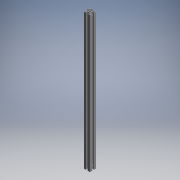
# Autodesk Inventor part: NFS5-2020-437-Z6-XA10-XB427
Saved by Autodesk Inventor 2017.3 (Build 213256000, 256)
## iProperties
Part Number: NFS5-2020-437-Z6-XA10-XB427
Material: Generic
Catalog Web Link: www.cadenas.de
Description: NFS5-2020, NFSB5-2020, HFS5-2020, HFSB5-2020, CAF5-2020, HFSY5-2020, NFSF5-2020, HFSF5-2020, HFSFB5-2020, NFST5-2020, HFST5-2020, HFSTB5-2020, HFSH5-2020, HFSC5-2020-HFS5 Series Aluminum Extrusions 20 Square -1 Slot-
Vendor: MISUMI
Document SubType Name: Modeling
Designer: partserver
Manufacturer: MISUMI
Mass: 78.6573 g
Surface Area: 763.15 cm^2
Volume: 78.6573 cm^3
Density: 1 g/cm^3
Appearance: PSOLRGB-175-175-175
Category: PARTsolutions
Company: MISUMI
Title: NFS5-2020-437-Z6-XA10-XB427
Author: Cadenas PARTsolutions
Comments: HFS5 Series Aluminum Extrusions 20 Square -1 Slot-
PSOL_IDENT_0: {$CADENAS_DATA\23d-libs\misumi\metric\38_al_extrusions_blackets\5\hfs5_2020.prj},704 {VTYP=3D},{NB=N
PSOL_IDENT_1: FS5-2020-437-Z6-XA10-XB427},{LINA=NFS5-2020-437-Z6-XA10-XB427},{NN=NFS5-2020, NFSB5-2020, HFS5-2020,
PSOL_IDENT_2: HFSB5-2020, CAF5-2020, HFSY5-2020, NFSF5-2020, HFSF5-2020, HFSFB5-2020, NFST5-2020, HFST5-2020, HFS
PSOL_IDENT_3: TB5-2020, HFSH5-2020, HFSC5-2020},{DATE=09.09.2019 15:28:27},{GEOMDATE=18.06.2019 07:59:14},{VERSION=
PSOL_IDENT_4: },{LINEID=10},{WBVAR=L,ALT1,ALT2,ALT4,ALT5,CP5,DL5,DR5,ALT6,ALT9,ALT10,ALT11,HP6,NHL6,DL6,NHR6,DR6,A
PSOL_IDENT_5: LT7,ALT8,NH9,AH,BH,CH,DH,EH,NH10,AV,BV,CV,DV,EV,NH11,AP,BP,CP,DP,EP,ALT12,ALT13,Z,NH12,XA,XB,XC,XD,X
PSOL_IDENT_6: E,NH13,YA,YB,YC,YD,YE,ALT16,HP16,DL16,DR16,ALT17,HQ17,JLP,ALT20},{WBNUMERIC=L,NH9,AH,BH,CH,DH,EH,NH1
PSOL_IDENT_7: 0,AV,BV,CV,DV,EV,NH11,AP,BP,CP,DP,EP,NH12,XA,XB,XC,XD,XE,NH13,YA,YB,YC,YD,YE,HQ17,JLP}  {NB=NFS5-202
PSOL_IDENT_8: 0-437-Z6-XA10-XB427},{LINA=NFS5-2020-437-Z6-XA10-XB427},{KT=DUMMY},{PN=NFS5-2020-437-Z6-XA10-XB427},
PSOL_IDENT_9: {TPS=NFS5-2020},{MAT=6063-T5 Aluminum Alloy},{ST=Clear Anodize},{FRMW=20},{FRMH=20},{FRD=4.2},{L=437
PSOL_IDENT_10: },{MASS=0.5},{SA=183},{LX=0.742x10^4},{LY=0.742x10^4},{ALT1=},{M1=0},{DPL1=0},{DPR1=0},{ALT1PN=},{AL
PSOL_IDENT_11: T2=},{ALT2ALG= '','w/o End Tapping (Heli-Coil Insert)','LHP','with LHP (Tapping on the Left (Heli-Co
PSOL_IDENT_12: il Insert))','RHP','with RHP (Tapping on the Right (Heli-Coil Insert))','HPW','with HPW (Tapping on
PSOL_IDENT_13: Both Ends (Heli-Coil Insert))' },{M2=0},{DP2=0},{ALT2PN=},{ALT4=},{ALT4ALG= '', 'w/o SC (High Precis
PSOL_IDENT_14: ion Cut)', 'SC', 'with SC (High Precision Cut)' },{ALT4PN=},{ALT5=},{ALT5ALG= '','w/o 45 Degree Cut'
PSOL_IDENT_15: ,'1','with 45 Degree Cut' },{CP5=},{CP5ALG= '','N/A' },{DL5=},{DL5ALG= '','N/A' },{DR5=},{DR5ALG= ''
PSOL_IDENT_16: ,'N/A' },{FRMLALT5=0},{FRMRALT5=0},{ALT5PN=},{ALT6=},{ALT6ALG= '','w/o Fastening Location Wrench Acc
PSOL_IDENT_17: ess Hole Alterations','1','with Fastening Location Wrench Access Hole Alterations' },{ALT9=},{ALT9AL
PSOL_IDENT_18: G= '','w/o Location Specified Wrench Access Hole Alteratons (Horizontal)','1','with Location Specifi
PSOL_IDENT_19: ed Wrench Access Hole Alteratons (Horizontal)' },{ALT10=},{ALT10ALG= '','w/o Location Specified Wren
PSOL_IDENT_20: ch Access Hole Alteratons (Vertical)','1','with Location Specified Wrench Access Hole Alteratons (Ve
PSOL_IDENT_21: rtical)' },{ALT11=},{ALT11ALG= '','w/o Location Specified Wrench Access Hole Alteratons (Crisscross)'
PSOL_IDENT_22: ,'1','with Location Specified Wrench Access Hole Alteratons (Crisscross)' },{HP6=},{HP6ALG= '','N/A'
PSOL_IDENT_23: },{NHL6=},{NHL6ALG= '','N/A' },{DL6=},{DL6ALG= '','N/A' },{NHR6=},{NHR6ALG= '','N/A' },{DR6=},{DR6A
PSOL_IDENT_24: LG= '','N/A' },{HL6=0.000},{HL6D=0},{HR6=0.000},{HR6D=0},{J6=0},{J6D=0},{K6=0},{K6D=0},{DD6=0.00},{D
PSOL_IDENT_25: D6ALG=0},{ALT7=},{ALT7ALG= '','N/A' },{ALT8=},{ALT8ALG= '','N/A' },{ALT678PN=},{NH9=0},{NH9MAX=5},{N
PSOL_IDENT_26: H9ALG=[0]},{AH=0.0},{AHMIN=7},{AHMAX=432},{AHALG=[0]},{BH=0.0},{BHMIN=2},{BHMAX=434},{BHALG=[0]},{CH=
PSOL_IDENT_27: 0.0},{CHMIN=2},{CHMAX=436},{CHALG=[0]},{DH=0.0},{DHMIN=2},{DHMAX=438},{DHALG=[0]},{EH=0.0},{EHMIN=2}
PSOL_IDENT_28: ,{EHMAX=430},{EHALG=[0]},{NH10=0},{NH10MAX=5},{NH10ALG=[0]},{AV=0.0},{AVMIN=7},{AVMAX=432},{AVALG=[0
PSOL_IDENT_29: ]},{BV=0.0},{BVMIN=2},{BVMAX=434},{BVALG=[0]},{CV=0.0},{CVMIN=2},{CVMAX=436},{CVALG=[0]},{DV=0.0},{D
PSOL_IDENT_30: VMIN=2},{DVMAX=438},{DVALG=[0]},{EV=0.0},{EVMIN=2},{EVMAX=430},{EVALG=[0]},{NH11=0},{NH11MAX=5},{NH1
PSOL_IDENT_31: 1ALG=[0]},{AP=0.0},{APMIN=7},{APMAX=432},{APALG=[0]},{BP=0.0},{BPMIN=2},{BPMAX=434},{BPALG=[0]},{CP=
PSOL_IDENT_32: 0.0},{CPMIN=2},{CPMAX=436},{CPALG=[0]},{DP=0.0},{DPMIN=2},{DPMAX=438},{DPALG=[0]},{EP=0.0},{EPMIN=2}
PSOL_IDENT_33: ,{EPMAX=430},{EPALG=[0]},{ALT9PN=},{ALT10PN=},{ALT11PN=},{ALT91011PN=},{ALT12=1},{ALT12ALG= '','w/o
PSOL_IDENT_34: Counterbore Hole in Specified Position (Vertical)','1','with Counterbore Hole in Specified Position
PSOL_IDENT_35: (Vertical)' },{ALT13=},{ALT13ALG= '','w/o Counterbore Hole in Specified Position (Horizontal)','1','
PSOL_IDENT_36: with Counterbore Hole in Specified Position (Horizontal)' },{Z=6},{ZALG='5','5','6','6'},{DD12=6.5},
PSOL_IDENT_37: {DD112=11.0},{NH12=2},{NH12MAX=5},{NH12ALG=[1:5/1]},{XA=10.0},{XAMIN=7},{XAMAX=417},{XAALG=[7:417/0.
PSOL_IDENT_38: 5]},{XB=427.0},{XBMIN=23},{XBMAX=430},{XBALG=[23:430/0.5]},{XC=0.0},{XCMIN=440},{XCMAX=443},{XCALG=[
PSOL_IDENT_39: 0]},{XD=0.0},{XDMIN=13},{XDMAX=456},{XDALG=[0]},{XE=0.0},{XEMIN=13},{XEMAX=430},{XEALG=[0]},{NH13=0}
PSOL_IDENT_40: ,{NH13MAX=5},{NH13ALG=[0]},{YA=0.0},{YAMIN=7},{YAMAX=443},{YAALG=[0]},{YB=0.0},{YBMIN=13},{YBMAX=456
PSOL_IDENT_41: },{YBALG=[0]},{YC=0.0},{YCMIN=13},{YCMAX=469},{YCALG=[0]},{YD=0.0},{YDMIN=13},{YDMAX=482},{YDALG=[0]
PSOL_IDENT_42: },{YE=0.0},{YEMIN=13},{YEMAX=430},{YEALG=[0]},{ALT12PN=-XA10-XB427},{ALT13PN=},{ALT1213PN=-Z6-XA10-X
PSOL_IDENT_43: B427},{ALT16=},{ALT16ALG= '','w/o M Type Hole Alteration','1','with M Type Hole Alteration' },{HP16=
PSOL_IDENT_44: },{HP16ALG= '','N/A' },{DL16=},{DL16ALG= '','N/A' },{DR16=},{DR16ALG= '','N/A' },{H116=0},{D16=0.0},
PSOL_IDENT_45: {ALT16PN=},{ALT17=},{ALT17ALG= '','w/o L Type Hole Alteration (Top)','1','with L Type Hole Alteratio
PSOL_IDENT_46: n (Top)' },{HQ17=0},{HQ17ALG=0},{JLP=0},{JLPMIN=4.9},{JLPMAX=0},{JLPALG=[0]},{L17=0},{D17=0.0},{ALT1
PSOL_IDENT_47: 7PN=},{ALT20=},{ALT20PN=},{ERRORALT01=OK},{ERRORALT02=OK},{ERRORALT05=OK},{ERRORALT06091=OK},{ERRORA
PSOL_IDENT_48: LT06092=OK},{ERRORALT06093=OK},{ERRORALT06094=OK},{ERRORALT06101=OK},{ERRORALT06102=OK},{ERRORALT061
PSOL_IDENT_49: 03=OK},{ERRORALT06104=OK},{ERRORALT06111=OK},{ERRORALT06112=OK},{ERRORALT06113=OK},{ERRORALT06114=OK
PSOL_IDENT_50: },{ERRORALT06121=OK},{ERRORALT06122=OK},{ERRORALT06123=OK},{ERRORALT06124=OK},{ERRORALT06131=OK},{ER
PSOL_IDENT_51: RORALT06132=OK},{ERRORALT06133=OK},{ERRORALT06134=OK},{ERRORALT0616=OK},{ERRORALT06171=OK},{ERRORALT
PSOL_IDENT_52: 06172=OK},{ERRORALT06173=OK},{ERRORALT0911=OK},{ERRORALT0913=OK},{ERRORALT0916=OK},{ERRORALT0917=OK}
PSOL_IDENT_53: ,{ERRORALT1011=OK},{ERRORALT1012=OK},{ERRORALT1016=OK},{ERRORALT1017=OK},{ERRORALT1112=OK},{ERRORALT
PSOL_IDENT_54: 1113=OK},{ERRORALT1116=OK},{ERRORALT1117=OK},{ERRORALT1216=OK},{ERRORALT1217=OK},{ERRORALT1316=OK},{
PSOL_IDENT_55: ERRORALT1317=OK},{ERRORALT1617=OK},{ERRORPN=},{TFW=0}
NB: NFS5-2020-437-Z6-XA10-XB427
NN: NFS5-2020, NFSB5-2020, HFS5-2020, HFSB5-2020, CAF5-2020, HFSY5-2020, NFSF5-2020, HFSF5-2020, HFSFB5-2020, NFST5-2020, HFST5-2020, HFSTB5-2020, HFSH5-2020, HFSC5-2020
NT: HFS5 Series Aluminum Extrusions 20 Square -1 Slot-
NBSYN: $PN.
LINA: NFS5-2020-437-Z6-XA10-XB427
CATALOG: Misumi
PN: NFS5-2020-437-Z6-XA10-XB427
TPS: NFS5-2020
MAT: 6063-T5 Aluminum Alloy
ST: Clear Anodize
L: 437
MASS: 0.5
SA: 183
LX: 0.742x10^4
LY: 0.742x10^4
ALT1: w/o End Tapping
M1: 0
DPL1: 0
DPR1: 0
ALT2: w/o End Tapping (Heli-Coil Insert)
M2: 0
DP2: 0
ALT4: w/o SC (High Precision Cut)
ALT5: w/o 45 Degree Cut
CP5: N/A
DL5: N/A
DR5: N/A
ALT6: w/o Fastening Location Wrench Access Hole Alterations
ALT9: w/o Location Specified Wrench Access Hole Alteratons (Horizontal)
ALT10: w/o Location Specified Wrench Access Hole Alteratons (Vertical)
ALT11: w/o Location Specified Wrench Access Hole Alteratons (Crisscross)
HP6: N/A
NHL6: N/A
DL6: N/A
NHR6: N/A
DR6: N/A
HL6D: 0
HR6D: 0
J6D: 0
K6D: 0
DD6: 0
ALT7: N/A
ALT8: N/A
NH9: 0
AH: 0
BH: 0
CH: 0
DH: 0
EH: 0
NH10: 0
AV: 0
BV: 0
CV: 0
DV: 0
EV: 0
NH11: 0
AP: 0
BP: 0
CP: 0
DP: 0
EP: 0
ALT12: with Counterbore Hole in Specified Position (Vertical)
ALT13: w/o Counterbore Hole in Specified Position (Horizontal)
Z: 6
DD12: 6.5
DD112: 11
NH12: 2
XA: 10
XB: 427
XC: 0
XD: 0
XE: 0
NH13: 0
YA: 0
YB: 0
YC: 0
YD: 0
YE: 0
ALT16: w/o M Type Hole Alteration
HP16: N/A
DL16: N/A
DR16: N/A
H116: 0
D16: 0
ALT17: w/o L Type Hole Alteration (Top)
HQ17: 0
JLP: 0
D17: 0
ALT20: w/o CW (End Face C Chamfering)
SUPPLIER: MISUMI
ARTICLENO: NFS5-2020-437-Z6-XA10-XB427
BOMINFO: NFS5-2020-437-Z6-XA10-XB427
CREATOR: CADENAS GmbH
Autodesk Inventor part; units mm, degrees
sketch "Sketch_75" plane through (0, 0, 0) normal (0, 0, 1) x (1, 0, 0)
  line L0 (-10, -3) -> (-10, -9)
  arc A0 (-10, -9) -> (-9, -10) centre (-9, -9) ccw
  line L1 (-9, -10) -> (-3, -10)
  line L2 (-3, -10) -> (-3, -8)
  line L3 (-3, -8) -> (-6, -8)
  line L4 (-6, -8) -> (-6, -7.0607)
  line L5 (-6, -7.0607) -> (-2.9393, -4)
  line L6 (-2.9393, -4) -> (-0.6536, -4)
  arc A1 (-0.6536, -4) -> (-0.4036, -3.933) centre (-0.6536, -3.5) ccw
  line L7 (-0.4036, -3.933) -> (0, -3.7)
  line L8 (0, -3.7) -> (0.4036, -3.933)
  arc A2 (0.4036, -3.933) -> (0.9036, -3.933) centre (0.6536, -3.5) ccw
  line L9 (0.9036, -3.933) -> (1.2189, -3.751)
  line L10 (1.2189, -3.751) -> (2.5, -4)
  line L11 (2.5, -4) -> (2.9393, -4)
  line L12 (2.9393, -4) -> (6, -7.0607)
  line L13 (6, -7.0607) -> (6, -8)
  line L14 (6, -8) -> (3, -8)
  line L15 (3, -8) -> (3, -10)
  line L16 (3, -10) -> (9, -10)
  arc A3 (9, -10) -> (10, -9) centre (9, -9) ccw
  line L17 (10, -9) -> (10, -3)
  line L18 (10, -3) -> (8, -3)
  line L19 (8, -3) -> (8, -6)
  line L20 (8, -6) -> (7.0607, -6)
  line L21 (7.0607, -6) -> (4, -2.9393)
  line L22 (4, -2.9393) -> (4, -0.6536)
  arc A4 (4, -0.6536) -> (3.933, -0.4036) centre (3.5, -0.6536) ccw
  line L23 (3.933, -0.4036) -> (3.7, 0)
  line L24 (3.7, 0) -> (3.933, 0.4036)
  arc A5 (3.933, 0.4036) -> (3.933, 0.9036) centre (3.5, 0.6536) ccw
  line L25 (3.933, 0.9036) -> (3.751, 1.2189)
  line L26 (3.751, 1.2189) -> (4, 2.5)
  line L27 (4, 2.5) -> (4, 2.9393)
  line L28 (4, 2.9393) -> (7.0607, 6)
  line L29 (7.0607, 6) -> (8, 6)
  line L30 (8, 6) -> (8, 3)
  line L31 (8, 3) -> (10, 3)
  line L32 (10, 3) -> (10, 9)
  arc A6 (10, 9) -> (9, 10) centre (9, 9) ccw
  line L33 (9, 10) -> (3, 10)
  line L34 (3, 10) -> (3, 8)
  line L35 (3, 8) -> (6, 8)
  line L36 (6, 8) -> (6, 7.0607)
  line L37 (6, 7.0607) -> (2.9393, 4)
  line L38 (2.9393, 4) -> (0.6536, 4)
  arc A7 (0.6536, 4) -> (0.4036, 3.933) centre (0.6536, 3.5) ccw
  line L39 (0.4036, 3.933) -> (0, 3.7)
  line L40 (0, 3.7) -> (-0.4036, 3.933)
  arc A8 (-0.4036, 3.933) -> (-0.9036, 3.933) centre (-0.6536, 3.5) ccw
  line L41 (-0.9036, 3.933) -> (-1.2189, 3.751)
  line L42 (-1.2189, 3.751) -> (-2.5, 4)
  line L43 (-2.5, 4) -> (-2.9393, 4)
  line L44 (-2.9393, 4) -> (-6, 7.0607)
  line L45 (-6, 7.0607) -> (-6, 8)
  line L46 (-6, 8) -> (-3, 8)
  line L47 (-3, 8) -> (-3, 10)
  line L48 (-3, 10) -> (-9, 10)
  arc A9 (-9, 10) -> (-10, 9) centre (-9, 9) ccw
  line L49 (-10, 9) -> (-10, 3)
  line L50 (-10, 3) -> (-8, 3)
  line L51 (-8, 3) -> (-8, 6)
  line L52 (-8, 6) -> (-7.0607, 6)
  line L53 (-7.0607, 6) -> (-4, 2.9393)
  line L54 (-4, 2.9393) -> (-4, 0.6536)
  arc A10 (-4, 0.6536) -> (-3.933, 0.4036) centre (-3.5, 0.6536) ccw
  line L55 (-3.933, 0.4036) -> (-3.7, 0)
  line L56 (-3.7, 0) -> (-3.933, -0.4036)
  arc A11 (-3.933, -0.4036) -> (-3.933, -0.9036) centre (-3.5, -0.6536) ccw
  line L57 (-3.933, -0.9036) -> (-3.751, -1.2189)
  line L58 (-3.751, -1.2189) -> (-4, -2.5)
  line L59 (-4, -2.5) -> (-4, -2.9393)
  line L60 (-4, -2.9393) -> (-7.0607, -6)
  line L61 (-7.0607, -6) -> (-8, -6)
  line L62 (-8, -6) -> (-8, -3)
  line L63 (-8, -3) -> (-10, -3)
  constraints: 128 end point, 24 point on circle, 12 centre point
extrude "Extrusion1" add sketch "Sketch_75" against normal blind 437
sketch "Sketch2" plane through (0, 0, -437) normal (0, 0, -1) x (-1, 0, 0)
  point P0 (0, 0)
hole "Hole1" at (0, 0, -437) direction (0, 0, 1) diameter 4.2 depth 437
sketch "Sketch_30" plane through (0, 0, 0) normal (1, 0, 0) x (0, 0, -1)
  line L0 (10, -10) -> (10, 10)
  line L1 (10, 10) -> (15.5, 10)
  line L2 (15.5, 10) -> (15.5, 4)
  line L3 (15.5, 4) -> (13.25, 4)
  line L4 (13.25, 4) -> (13.25, -10)
  line L5 (13.25, -10) -> (10, -10)
  line L6 (10, -10) -> (10, 10)
  constraints: 14 end point
revolve "Revolution1" cut sketch "Sketch_30" angle 360 about axis through (0, -10, -10) along (0, -1, 0)
sketch "Sketch_31" plane through (0, 0, 0) normal (1, 0, 0) x (0, 0, -1)
  line L0 (427, -10) -> (427, 10)
  line L1 (427, 10) -> (432.5, 10)
  line L2 (432.5, 10) -> (432.5, 4)
  line L3 (432.5, 4) -> (430.25, 4)
  line L4 (430.25, 4) -> (430.25, -10)
  line L5 (430.25, -10) -> (427, -10)
  line L6 (427, -10) -> (427, 10)
  constraints: 14 end point
revolve "Revolution2" cut sketch "Sketch_31" angle 360 about axis through (0, -10, -427) along (0, -1, 0)
ref_plane "C1_XY" through (0, 0, 0) normal (0, 0, 1) x (1, 0, 0)
ref_plane "C1_YZ" through (0, 0, 0) normal (1, 0, 0) x (0, 1, 0)
ref_plane "C1_ZX" through (0, 0, 0) normal (0, 1, 0) x (0, 0, 1)
body "Solid1"
